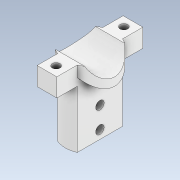
# Autodesk Inventor part: soporte_flauta_3
Saved by Autodesk Inventor 2022 (Build 260153000, 153)
## iProperties
Created: 2022-05-10
Part Number: soporte_flauta_3
Material: Generic
Document SubType Name: Modeling
Designer: ferna
Density: 1 g/cm^3
Appearance: Snow
Author: ferna
Autodesk Inventor part; units mm, degrees
ref_plane "YZ Plane" through (0, 0, 0) normal (1, 0, 0) x (0, 1, 0)
sketch "Sketch1" plane through (0, 0, 0) normal (0, 1, 0) x (-1, 0, 0)
  circle A0 centre (0, 0) radius 14
  circle A1 centre (0, 0) radius 11
  dimension "d0" = 28
  dimension "d1" = 22
  constraints: 2 centre point, 2 coincident
  measures "d0" diameter of A0
  measures "d1" diameter of A1
extrude "Extrusion1" add sketch "Sketch1" along normal blind 10
sketch "Sketch2" plane through (0, 10, 0) normal (0, 1, 0) x (1, 0, 0)
  circle A0 centre (0, 0) radius 17.5
  dimension "d4" = 35
  constraints: 1 centre point, 1 coincident
  measures "d4" diameter of A0
extrude "Extrusion2" add sketch "Sketch2" along normal blind 3
sketch "Sketch3" plane through (0, 0, 0) normal (1, 0, 0) x (0, 1, 0)
  line L0 (13, -17.5) -> (13, 17.5) projected
  line L1 (13, 0) -> (28, 0)
  circle A0 centre (28, 0) radius 15
  line L2 (28, -15) -> (28, -17.5)
  line L3 (28, -17.5) -> (13, -17.5)
  line L4 (13, -17.5) -> (13, 17.5)
  line L5 (13, 17.5) -> (28, 17.5)
  line L6 (10, 17.5) -> (13, 17.5) projected
  line L7 (28, 17.5) -> (28, 15)
  point P0 (0, 0)
  dimension "d7" = 15
  constraints: 12 end point, 3 point on circle, 2 collinear, 2 point on line, 1 centre point, 1 coincident, 1 horizontal, 1 midpoint, 1 perpendicular, 1 vertical
  measures "d7" distance of L1.start L1.end
extrude "Extrusion3" add sketch "Sketch3" along normal up to surface contours L0 A0 L2 L3 | L0 L5 L7 A0 round surface about axis through (0, 10, 0) along (0, 1, 0) radius 17.5 far side no
sketch "Sketch4" plane through (0, 0, 0) normal (-1, 0, 0) x (0, 0, 1)
  line L0 (-17.5, 28) -> (-15, 28) projected
  line L1 (-17.5, 13) -> (-17.5, 28) projected
  line L2 (0, 13) -> (-17.5, 13) projected
  arc A0 (-15, 28) -> (0, 13) centre (0, 28) ccw projected
  line L3 (17.5, 13) -> (0, 13) projected
  line L4 (17.5, 13) -> (17.5, 28) projected
  line L5 (15, 28) -> (17.5, 28) projected
  arc A1 (0, 13) -> (15, 28) centre (0, 28) ccw projected
  point P0 (0, 0)
extrude "Extrusion4" add sketch "Sketch4" along normal up to surface round surface about axis through (0, 10, 0) along (0, 1, 0) radius 17.5 far side no
sketch "Sketch5" plane through (0, 0, 0) normal (0, 0, 1) x (1, 0, 0)
  line L0 (-9.0139, 28) -> (9.0139, 28) projected
  line L1 (0, 28) -> (0, 25)
  line L2 (0, 25) -> (5, 25)
  line L3 (5, 25) -> (5, 23)
  line L4 (5, 23) -> (-5, 23)
  line L5 (-5, 23) -> (-5, 25)
  line L6 (-5, 25) -> (0, 25)
  point P0 (0, 0)
  dimension "d12" = 3
  dimension "d13" = 5
  dimension "d14" = 2
  dimension "d15" = 10
  constraints: 12 end point, 5 perpendicular, 1 midpoint, 1 point on line, 1 vertical
  measures "d12" distance of L1.start L1.end
  measures "d13" distance of L1.end L2.end
  measures "d14" distance of L2.end L3.end
  measures "d15" distance of L3.end L4.end
extrude "Extrusion5" cut sketch "Sketch5" along normal through all both and the other way through all
sketch "Sketch6" plane through (0, 10, 0) normal (0, -1, 0) x (1, 0, 0)
  circle A0 centre (0, 0) radius 14 projected
  circle A1 centre (0, 0) radius 14.5
  dimension "d18" = 29
  constraints: 1 centre point, 1 coincident
  measures "d18" diameter of A1
extrude "Extrusion6" add sketch "Sketch6" along normal up to surface (10 mm away)
ref_plane "Work Plane1" through (0, 25, 17.5) normal (0, 0, 1) x (1, 0, 0)
sketch "Sketch7" plane through (0, 25, 17.5) normal (0, 0, 1) x (1, 0, 0)
  line L0 (5, -2) -> (-5, -2) projected
  line L1 (5, -2) -> (13.7117, -2)
  line L2 (13.7117, -2) -> (0, 13.5732)
  line L3 (0, 13.5732) -> (-17.6873, -2)
  line L4 (-17.6873, -2) -> (5, -2)
  point P0 (0, -25)
  constraints: 8 end point, 1 collinear, 1 horizontal, 1 perpendicular, 1 point on line
extrude "Extrusion7" cut sketch "Sketch7" against normal through all
sketch "Sketch8" plane through (0, 25, 17.5) normal (0, 0, 1) x (1, 0, 0)
  line L0 (-10.3078, -2) -> (10.3078, -2) projected
  line L1 (-10.3078, -2) -> (10.3078, -2) projected
  line L2 (17.5, -12) -> (-17.5, -12) projected
  line L3 (-10.3078, -2) -> (10.3078, -2)
  line L4 (10.3078, -2) -> (10.3078, -12)
  line L5 (10.3078, -12) -> (-10.3078, -12)
  line L6 (-10.3078, -12) -> (-10.3078, -2)
  line L7 (17.5, -12) -> (-17.5, -12)
  line L8 (-17.5, -12) -> (-17.5, -2)
  line L9 (-17.5, -2) -> (17.5, -2)
  line L10 (17.5, -2) -> (17.5, -12)
  line L11 (-11, -15) -> (11, -15) projected
  line L12 (-10.3078, -12) -> (10.3078, -12)
  line L13 (10.3078, -12) -> (10.3078, -15)
  line L14 (10.3078, -15) -> (-10.3078, -15)
  line L15 (-10.3078, -15) -> (-10.3078, -12)
  point P0 (0, -25)
  constraints: 24 end point, 6 parallel, 3 horizontal, 3 perpendicular, 3 point on line
extrude "Extrusion8" add sketch "Sketch8" along normal up to surface contours L0 L4 L2 L6 | L2 L13 L11 L15 round surface about axis through (0, 10, 0) along (0, 1, 0) radius 17.5 far side no
sketch "Sketch9" plane through (0, 25, 17.5) normal (0, 0, 1) x (1, 0, 0)
  line L0 (10.3078, -2) -> (-10.3078, -2) projected
  line L1 (-10.3078, -2) -> (-10.3078, -15) projected
  line L2 (-10.3078, -15) -> (10.3078, -15) projected
  line L3 (10.3078, -15) -> (10.3078, -2) projected
  point P0 (0, -25)
extrude "Extrusion9" add sketch "Sketch9" along normal blind 13
ref_plane "Work Plane2" through (0, 10, -17.5) normal (0, 0, 1) x (1, 0, 0)
sketch "Sketch12" plane through (0, 10, -17.5) normal (0, 0, 1) x (1, 0, 0)
  line L0 (-10.3078, 13) -> (-10.3078, 0) projected
  line L1 (10.3078, 13) -> (-10.3078, 13) projected
  line L2 (-10.3078, 0) -> (10.3078, 0) projected
  line L3 (10.3078, 0) -> (10.3078, 13) projected
  point P0 (0, -10)
extrude "Extrusion12" add sketch "Sketch12" along normal up to surface round surface about axis through (0, 10, 0) along (0, 1, 0) radius 17.5 far side no
sketch "Sketch13" plane through (0, 10, -17.5) normal (0, 0, -1) x (-1, 0, 0)
  line L0 (-10.3078, 13) -> (10.3078, 13) projected
  line L1 (10.3078, 13) -> (10.3078, 0) projected
  line L2 (-10.3078, 0) -> (-10.3078, 13) projected
  line L3 (10.3078, 0) -> (-10.3078, 0) projected
  point P0 (0, -10)
extrude "Extrusion13" add sketch "Sketch13" along normal blind 13
sketch "Sketch17" plane through (0, 10, 0) normal (0, -1, 0) x (1, 0, 0)
  circle A0 centre (0, 0) radius 17.5
  line L0 (0, -17.5) -> (0, -30.5)
  line L1 (-10.3078, -30.5) -> (10.3078, -30.5)
  line L2 (-4.9075, 24) -> (-2.4537, 28.25)
  line L3 (-2.4537, 19.75) -> (-4.9075, 24)
  line L4 (2.4537, 19.75) -> (-2.4537, 19.75)
  line L5 (4.9075, 24) -> (2.4537, 19.75)
  line L6 (2.4537, 28.25) -> (4.9075, 24)
  line L7 (-2.4537, 28.25) -> (2.4537, 28.25)
  circle A1 centre (0, 24) radius 2.75
  line L8 (-4.9075, -24) -> (-2.4537, -19.75)
  line L9 (-2.4537, -28.25) -> (-4.9075, -24)
  line L10 (2.4537, -28.25) -> (-2.4537, -28.25)
  line L11 (4.9075, -24) -> (2.4537, -28.25)
  line L12 (2.4537, -19.75) -> (4.9075, -24)
  line L13 (-2.4537, -19.75) -> (2.4537, -19.75)
  circle A2 centre (0, -24) radius 2.75
  constraints: 28 end point, 2 centre point, 2 midpoint, 1 vertical alignment, 2 other
extrude "Extrusion16" cut sketch "Sketch17" against normal blind 2.8 contours L13 L12 L11 L10 L0 A2 | L0 A2 L10 L9 L8 L13 | L2 L7 L6 L5 L4 L3
sketch "Sketch18" plane through (0, 10, 0) normal (0, -1, 0) x (1, 0, 0)
  circle A0 centre (0, -24) radius 2.75 projected
  circle A1 centre (0, 24) radius 2.75 projected
  point P0 (0, 0)
extrude "Extrusion17" cut sketch "Sketch18" against normal through all
sketch "Sketch20" plane through (0, 0, 0) normal (0, -1, 0) x (1, 0, 0)
  circle A0 centre (0, 0) radius 14.5 projected
  circle A1 centre (0, 0) radius 11 projected
extrude "Extrusion18" add sketch "Sketch20" along normal blind 25
sketch "Sketch21" plane through (0, 10, 0) normal (0, -1, 0) x (1, 0, 0)
  arc A0 (-10.3078, 14.1421) -> (-10.3078, -14.1421) centre (0, 0) ccw projected
  circle A1 centre (0, 0) radius 11 projected
  circle A2 centre (0, 0) radius 17.5
  constraints: 1 centre point, 1 coincident
extrude "Extrusion19" add sketch "Sketch21" along normal blind 25
sketch "Sketch22" plane through (0, -25, 0) normal (0, -1, 0) x (1, 0, 0)
  circle A0 centre (0, 0) radius 12.8622
  constraints: 1 centre point, 1 coincident
extrude "Extrusion20" add sketch "Sketch22" against normal up to surface (35 mm away)
sketch "Sketch23" plane through (-10.3078, 23, 14.1421) normal (0, 1, 0) x (1, 0, 0)
  spline S0 degree 2 poles (-7.1922, 14.1421) (-7.1922, 5.2422) (0, 0) knots 0 0 0 1 1 1 weights 1 0.891352 1 projected
  spline S1 degree 2 poles (20.6155, 0) (27.8078, 5.2422) (27.8078, 14.1421) knots 0 0 0 1 1 1 weights 1 0.891352 1 projected
  circle A0 centre (10.3078, 14.1421) radius 17.5
  circle A1 centre (10.3078, 14.1421) radius 17.5 projected
  line L0 (10.3078, -3.3579) -> (3.3078, -3.3579)
  line L1 (3.3078, -3.3579) -> (3.3078, -18.248)
  line L2 (3.3078, -18.248) -> (-2.6812, -18.248)
  line L3 (-2.6812, -18.248) -> (-3.6117, 3.5357)
  line L4 (10.3078, -3.3579) -> (17.3078, -3.3579)
  line L5 (17.3078, -3.3579) -> (17.3078, -20.4363)
  line L6 (17.3078, -20.4363) -> (24.6729, -20.4363)
  line L7 (24.6729, -20.4363) -> (26.7802, 8.2336)
  arc A2 (20.6155, 28.2843) -> (0, 28.2843) centre (10.3078, 14.1421) ccw projected
  line L8 (10.3078, 31.6421) -> (17.3078, 31.6421)
  line L9 (17.3078, 31.6421) -> (17.3078, 48.9932)
  line L10 (17.3078, 48.9932) -> (24.6729, 48.9932)
  line L11 (24.6729, 48.9932) -> (24.6729, 24.1368)
  line L12 (10.3078, 31.6421) -> (3.3078, 31.6421)
  line L13 (3.3078, 31.6421) -> (3.3078, 53.0714)
  line L14 (3.3078, 53.0714) -> (-6.5605, 50.7837)
  line L15 (-6.5605, 50.7837) -> (-6.5605, 18.8019)
  line L16 (3.3078, -3.3579) -> (3.3078, -1.8969)
  line L17 (17.3078, -3.3579) -> (17.3078, -1.8969)
  line L18 (17.3078, 31.6421) -> (17.3078, 30.1812)
  line L19 (3.3078, 31.6421) -> (3.3078, 30.1812)
  point P0 (24.6729, 24.1368)
  point P1 (21.5813, 0.7572)
  point P2 (-0.9658, 0.7572)
  point P3 (-6.5605, 18.8019)
  point P4 (3.3078, 30.1812)
  dimension "d49" = 7
  dimension "d50" = 7
  dimension "d51" = 7
  dimension "d52" = 7
  constraints: 40 end point, 8 point on line, 6 perpendicular, 2 horizontal, 1 centre point, 1 coincident, 1 parallel, 1 point on circle, 1 tangent, 1 vertical, 14 other
  measures "d49" distance of L0.start L0.end
  measures "d50" distance of L0.start L4.end
  measures "d51" distance of L8.start L8.end
  measures "d52" distance of L8.start L12.end
extrude "Extrusion21" cut sketch "Sketch23" against normal through all contours S0 A0 L16 L1 L2 L3 | L15 L14 L13 L19 A0 | A0 S1 L7 L6 L5 L17 | L18 L9 L10 L11 A0
sketch "Sketch24" plane through (-7, 23, 16.039) normal (-1, 0, 0) x (0, 0, 1)
  circle A0 centre (-16.039, 0) radius 20
  line L0 (1.2815, -10) -> (7.3036, -55.1976)
  line L1 (7.3036, -55.1976) -> (-44.2958, -55.1976)
  line L2 (0, 0) -> (0, -13) projected
  line L3 (-44.2958, -55.1976) -> (-33.3595, -10)
  point P0 (-16.039, -23)
  point P1 (-20.6988, -9.2579)
  point P2 (-30.1812, 0)
  dimension "d55" = 40
  constraints: 6 end point, 2 point on circle, 1 centre point, 1 perpendicular
  measures "d55" diameter of A0
extrude "Extrusion22" cut sketch "Sketch24" along normal through all contours A0 L0 L1 L3
sketch "Sketch25" plane through (7, 23, -16.039) normal (1, 0, 0) x (0, 0, -1)
  circle A0 centre (-16.039, 0) radius 20
  line L0 (1.8461, -8.9512) -> (11.5805, -53.3288)
  line L1 (11.5805, -53.3288) -> (-49.8297, -54.5329)
  line L2 (-49.8297, -54.5329) -> (-33.9241, -8.9512)
  point P0 (-16.039, -23)
  point P1 (-16.039, -10)
  point P2 (-30.1812, 0)
  constraints: 6 end point, 2 point on circle, 1 centre point
extrude "Extrusion23" cut sketch "Sketch25" along normal through all contours A0 L0 L1 L2
sketch "Sketch26" plane through (7, 23, 30.5) normal (1, 0, 0) x (0, 0, -1)
  arc A0 (14.461, -11.9478) -> (46.539, -11.9478) centre (30.5, 0) ccw projected
  line L0 (30.5, -20) -> (30.5, -32.671)
  line L1 (30.5, -32.671) -> (30.5, -47.671)
  circle A1 centre (30.5, -32.671) radius 3
  circle A2 centre (30.5, -47.671) radius 3
  point P0 (30.5, -23)
  dimension "d60" = 12.671
  dimension "d61" = 15
  dimension "d62" = 6
  dimension "d63" = 6
  constraints: 4 end point, 2 centre point, 2 coincident, 1 point on circle, 1 point on line, 1 vertical
  measures "d60" distance of L0.start L0.end
  measures "d61" distance of L0.end L1.end
  measures "d62" diameter of A1
  measures "d63" diameter of A2
sketch "Sketch27" plane through (0, -25, 0) normal (0, -1, 0) x (1, 0, 0)
  line L0 (7, -16.039) -> (7, -12.6984) projected
  arc A0 (-7, -12.6984) -> (7, -12.6984) centre (0, 0) ccw projected
  line L1 (-7, -12.6984) -> (-7, -16.039) projected
  arc A1 (-7, -16.039) -> (7, -16.039) centre (0, 0) ccw projected
  line L2 (7, 12.6984) -> (7, 16.039) projected
  arc A2 (7, 16.039) -> (-7, 16.039) centre (0, 0) ccw projected
  line L3 (-7, 16.039) -> (-7, 12.6984) projected
  arc A3 (7, 12.6984) -> (-7, 12.6984) centre (0, 0) ccw projected
extrude "Extrusion24" add sketch "Sketch27" against normal up to surface (10 mm away)
sketch "Sketch28" plane through (0, -25, 0) normal (0, -1, 0) x (1, 0, 0)
  line L0 (7, -16.039) -> (7, 16.039) projected
  arc A0 (7, 16.039) -> (-7, 16.039) centre (0, 0) ccw projected
  line L1 (-7, 16.039) -> (-7, -16.039) projected
  arc A1 (-7, -16.039) -> (7, -16.039) centre (0, 0) ccw projected
extrude "Extrusion25" add sketch "Sketch28" along normal blind 10
extrude "Extrusion26" cut sketch "Sketch26" against normal through all
sketch "Sketch29" plane through (7, 23, 30.5) normal (1, 0, 0) x (0, 0, -1)
  circle A0 centre (30.5, 4.2388) radius 20
  line L0 (13, -5.4437) -> (10.5, -23)
  line L1 (10.5, -23) -> (57.7388, -23)
  line L2 (57.7388, -23) -> (48, -5.4437)
  line L3 (46.539, 0) -> (44.6421, 0) projected
  point P0 (30.5, -23)
  point P1 (30.5, 0)
  dimension "d70" = 40
  constraints: 6 end point, 2 horizontal alignment, 2 point on circle, 1 centre point, 1 horizontal, 2 other
  measures "d70" diameter of A0
extrude "Extrusion27" cut sketch "Sketch29" along normal through all contours A0 L2 L1 L0
sketch "Sketch30" plane through (-7, 23, -30.5) normal (-1, 0, 0) x (0, 0, 1)
  spline S0 degree 2 poles (46.539, -7.709) (30.5, -29.2402) (14.461, -7.709) knots 0 0 0 1 1 1 weights 1 0.59739 1 projected
  line L0 (14.461, -7.709) -> (5.7951, -19.3277)
  line L1 (5.7951, -19.3277) -> (57.7388, -24.3954)
  line L2 (46.539, 0) -> (46.539, -7.709) projected
  line L3 (57.7388, -24.3954) -> (46.539, -7.709)
  point P0 (30.5, -23)
  constraints: 6 end point, 1 horizontal alignment
extrude "Extrusion28" cut sketch "Sketch30" along normal through all
sketch "Sketch31" plane through (0, -35, 0) normal (0, -1, 0) x (1, 0, 0)
  arc A0 (7, 16.039) -> (-7, 16.039) centre (0, 0) ccw projected
  line L0 (-7, 16.039) -> (-7, -16.039) projected
  arc A1 (-7, -16.039) -> (7, -16.039) centre (0, 0) ccw projected
  line L1 (7, -16.039) -> (7, 16.039) projected
extrude "Extrusion29" cut sketch "Sketch31" against normal blind 4.329
body "Solid1"
